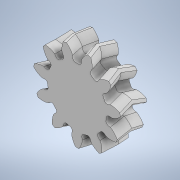
# Autodesk Inventor part: SmallGearV5
Saved by Autodesk Inventor 2022 (Build 260153070, 153G)
## iProperties
Created: 2022-01-26
Part Number: SmallGearV5
Material: Generic
Document SubType Name: Modeling
Designer: a laptop
Density: 1 g/cm^3
Appearance: Default
Author: a laptop
Autodesk Inventor part; units mm, degrees
ref_plane "YZ Plane" through (0, 0, 0) normal (1, 0, 0) x (0, 1, 0)
ref_plane "XZ Plane" through (0, 0, 0) normal (0, 1, 0) x (-1, 0, 0)
ref_plane "XY Plane" through (0, 0, 0) normal (0, 0, 1) x (1, 0, 0)
sketch "Sketch1" plane through (0, 0, 0) normal (0, 0, 1) x (1, 0, 0)
  spline S0 degree 3 poles (-1.222686, 4.833198) (-1.146742, 4.771577) (-0.994859, 4.64834) (-0.793987, 4.433475) (-0.650965, 4.234702) (-0.556471, 4.062893) (-0.524892, 3.97026) (-0.509107, 3.92396) knots 0 0 0 0 0.25004061 0.50007002 0.75001451 0.87505322 1 1 1 1
  spline S1 degree 3 poles (-0.509107, 3.92396) (-0.512505, 3.847818) (-0.517601, 3.733595) (-0.47769, 3.586522) (-0.426114, 3.484311) (-0.33957, 3.405574) (-0.189425, 3.364479) (0, 3.39922) (0.189425, 3.364479) (0.33957, 3.405574) (0.426114, 3.484311) (0.47769, 3.586522) (0.517601, 3.733595) (0.512505, 3.847818) (0.509107, 3.92396) knots 0 0 0 0 0.12504611 0.18758556 0.25001803 0.31238045 0.37474055 0.5 0.62525945 0.68761955 0.74998197 0.81241444 0.87495389 1 1 1 1
  spline S2 degree 3 poles (0.509107, 3.92396) (0.524892, 3.97026) (0.556471, 4.062893) (0.650965, 4.234702) (0.793987, 4.433475) (0.994859, 4.64834) (1.146742, 4.771577) (1.222686, 4.833198) knots 0 0 0 0 0.12494678 0.24998549 0.49992998 0.74995939 1 1 1 1
  circle A0 centre (0, 0) radius 3.385312 construction
  circle A1 centre (0, 0) radius 3.921018 construction
  circle A2 centre (0, 0) radius 3.985813 construction
  circle A3 centre (0, 0) radius 4.985455
  point P0 (-0.999344, 4.643331)
  point P1 (-0.798839, 4.429506)
  point P2 (-0.629016, 4.190707)
  point P3 (-0.560375, 4.06118)
  point P4 (-0.503728, 3.697256)
  point P5 (-0.474052, 3.587794)
  point P6 (-0.420251, 3.488174)
  point P7 (-0.33526, 3.413565)
  point P8 (-0.227104, 3.380528)
  point P9 (0, 3.385312)
  point P10 (0.227104, 3.380528)
  point P11 (0.33526, 3.413565)
  point P12 (0.420251, 3.488174)
  point P13 (0.474052, 3.587794)
  point P14 (0.503728, 3.697256)
  point P15 (0.560375, 4.06118)
  point P16 (0.629016, 4.190707)
  point P17 (0.798839, 4.429506)
  point P18 (0.999344, 4.643331)
  constraints: 4 centre point, 2 point on circle, 53 other
sketch "Sketch1 outline for Extrusion1" plane through (0, 0, 0) normal (0, 0, 1) x (1, 0, 0)
  circle A0 centre (0, 0) radius 4.985455
extrude "Extrusion1" add sketch "Sketch1 outline for Extrusion1" against normal blind 1.5
sketch "Sketch1 outline for Coil1" plane through (0, 0, 0) normal (0, 0, 1) x (1, 0, 0)
  arc A0 (1.222686, 4.833198) -> (-1.222686, 4.833198) centre (0, 0) ccw
  spline S0 degree 3 poles (0.509107, 3.92396) (0.524892, 3.97026) (0.556471, 4.062893) (0.650965, 4.234702) (0.793987, 4.433475) (0.994859, 4.64834) (1.146742, 4.771577) (1.222686, 4.833198) knots 0 0 0 0 0.12494678 0.24998549 0.49992998 0.74995939 1 1 1 1
  spline S1 degree 3 poles (-0.509107, 3.92396) (-0.512505, 3.847818) (-0.517601, 3.733595) (-0.47769, 3.586522) (-0.426114, 3.484311) (-0.33957, 3.405574) (-0.189425, 3.364479) (0, 3.39922) (0.189425, 3.364479) (0.33957, 3.405574) (0.426114, 3.484311) (0.47769, 3.586522) (0.517601, 3.733595) (0.512505, 3.847818) (0.509107, 3.92396) knots 0 0 0 0 0.12504611 0.18758556 0.25001803 0.31238045 0.37474055 0.5 0.62525945 0.68761955 0.74998197 0.81241444 0.87495389 1 1 1 1
  spline S2 degree 3 poles (-1.222686, 4.833198) (-1.146742, 4.771577) (-0.994859, 4.64834) (-0.793987, 4.433475) (-0.650965, 4.234702) (-0.556471, 4.062893) (-0.524892, 3.97026) (-0.509107, 3.92396) knots 0 0 0 0 0.25004061 0.50007002 0.75001451 0.87505322 1 1 1 1
coil "Coil1" sketch "Sketch1 outline for Coil1" operation cut axis through (0, 0, -10) along (0, 0, -1) pitch 93.468379 turns 0.016048 hand left
pattern_circular "Circular Pattern1" count 11 over 360 about axis through (0, 0, -10) along (0, 0, 1) of "Coil1"
mirror "Mirror1" about plane through (0, 4.370513, -1.5) normal (0, 0, -1) of "Extrusion1", "Coil1", "Circular Pattern1"
equation "\"d0\" = FaceWidth"
equation "\"Module\" = 0.7"
equation "\"PressureAngle\" = 10deg"
equation "\"UnitProfileClearance\" = 0.25"
equation "\"UnitRoundRadius\" = 0.3025"
equation "\"HeadDiameter\" = 9.97091"
equation "\"RootDiameter\" = 6.77062"
equation "\"BaseDiameter\" = 7.84204"
equation "\"PitchDiameter\" = 7.97163"
equation "\"FaceWidth\" = 1.5"
equation "\"HelixAngle\" = 15deg"
equation "\"UnitCorrection\" = 0.433274"
equation "\"UnitAddendumModification\" = 0.005215"
equation "\"CircularPitch\" = 2.27669"
equation "\"UnitBacklashShift\" = -0.041134"
equation "\"TotalToolShift\" = 0.2745"
equation "\"IsInternal\" = 0"
body "Solid1"
